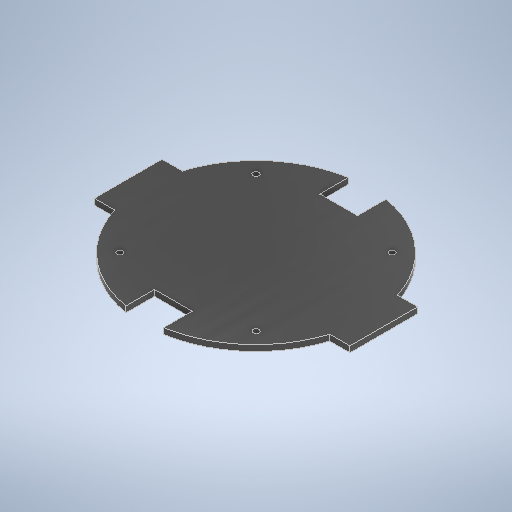
# Autodesk Inventor part: Base_inferior
Saved by Autodesk Inventor 2025.2 (Build 292293000, 293)
## iProperties
Created: 2025-11-06
Part Number: Base_inferior
Material: Genérico
Document SubType Name: Modeling
Designer: Dax
Density: 1 g/cm^3
Appearance: Gris oscuro
Author: Dax
Autodesk Inventor part; units mm, degrees
ref_plane "YZ Plane" through (0, 0, 0) normal (1, 0, 0) x (0, 1, 0)
ref_plane "XZ Plane" through (0, 0, 0) normal (0, 1, 0) x (-1, 0, 0)
ref_plane "XY Plane" through (0, 0, 0) normal (0, 0, 1) x (1, 0, 0)
sketch "Boceto1" plane through (0, 0, 0) normal (0, 1, 0) x (-1, 0, 0)
  line L0 (0, -55) -> (12.5, -55)
  line L1 (12.5, -55) -> (12.5, -73.951)
  line L2 (0, -55) -> (-12.5, -55)
  line L3 (-12.5, -55) -> (-12.5, -73.951)
  line L4 (0, 55) -> (12.5, 55)
  line L5 (12.5, 55) -> (12.5, 73.951)
  line L6 (0, 55) -> (-12.5, 55)
  line L7 (-12.5, 55) -> (-12.5, 73.951)
  line L8 (85, 0) -> (85, -22.5)
  line L9 (85, -22.5) -> (71.5454, -22.5)
  line L10 (85, 0) -> (85, 22.5)
  line L11 (85, 22.5) -> (71.5454, 22.5)
  line L12 (-85, 0) -> (-85, -22.5)
  line L13 (-85, -22.5) -> (-71.5454, -22.5)
  line L14 (-85, 0) -> (-85, 22.5)
  line L15 (-85, 22.5) -> (-71.5454, 22.5)
  arc A0 (12.5, -73.951) -> (71.5454, -22.5) centre (0, 0) ccw
  arc A1 (71.5454, 22.5) -> (12.5, 73.951) centre (0, 0) ccw
  arc A2 (-12.5, 73.951) -> (-71.5454, 22.5) centre (0, 0) ccw
  arc A3 (-71.5454, -22.5) -> (-12.5, -73.951) centre (0, 0) ccw
  dimension "d2" = 12.5
  dimension "d4" = 22.5
  constraints: 32 end point, 8 point on circle, 4 centre point, 2 perpendicular, 1 coincident
  measures "d2" distance of L0.start L0.end
  measures "d4" distance of L8.start L8.end
extrude "Extrusión1" add sketch "Boceto1" along normal blind 4
sketch "Boceto2" plane through (0, 4, 0) normal (0, 1, 0) x (1, 0, 0)
  circle A0 centre (0, 0) radius 64
  line L0 (0, 0) -> (64, 0) construction
  circle A1 centre (45.2548, 45.2548) radius 2
  circle A2 centre (-45.2548, 45.2548) radius 2
  circle A3 centre (-45.2548, -45.2548) radius 2
  circle A4 centre (45.2548, -45.2548) radius 2
  dimension "d9" = 4
  dimension "d12" = 360
  constraints: 5 centre point, 2 end point, 1 coincident, 1 horizontal, 9 other
  measures "d9" diameter of A1
extrude "Extrusión2" cut sketch "Boceto2" against normal blind 4 contours A1 A0 | A0 A1 | A4 A0 | A0 A4 | A2 A0 | A0 A2 | A3 A0 | A0 A3
